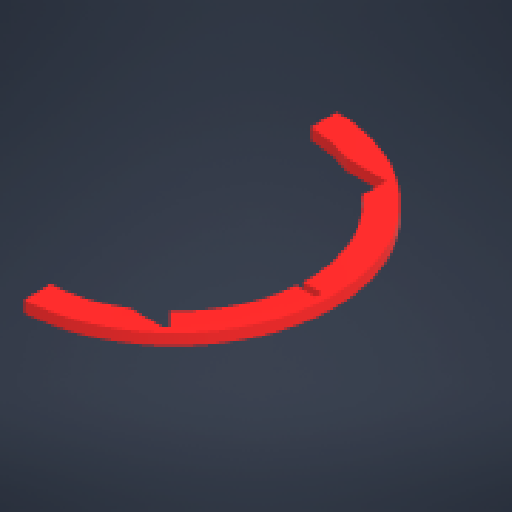
# Autodesk Inventor part: Back_front_aligner
Saved by Autodesk Inventor 2023 (Build 270158000, 158)
## iProperties
Created: 2023-05-09
Part Number: Back_front_aligner
Material: Generic
Document SubType Name: Modeling
Designer: szykr
Density: 1 g/cm^3
Appearance: Light Red
Author: szykr
Autodesk Inventor part; units mm, degrees
ref_plane "YZ Plane" through (0, 0, 0) normal (1, 0, 0) x (0, 1, 0)
ref_plane "XZ Plane" through (0, 0, 0) normal (0, 1, 0) x (-1, 0, 0)
ref_plane "XY Plane" through (0, 0, 0) normal (0, 0, 1) x (1, 0, 0)
sketch "Sketch1" plane through (0, 0, 0) normal (0, 1, 0) x (-1, 0, 0)
  circle A0 centre (0, 0) radius 40
  circle A1 centre (0, 0) radius 35
  line L0 (-0.75, -40) -> (-0.75, -35)
  line L1 (-23, -26.381812) -> (-23, -32.726136)
  line L2 (-34.93812, 2.828496) -> (-39.945867, 2.828496)
  line L3 (-39.945867, 1.33215) -> (-34.93812, 1.33215)
  line L4 (-24.132224, 25.315702) -> (-27.666452, 28.85856)
  line L5 (-26.660208, 29.866295) -> (-27.720868, 28.808219)
  line L6 (-39.940266, 2.933386) -> (-39.940266, 1.43704)
  line L7 (-23, -32.726136) -> (-21.5, -32.726136)
  circle A2 centre (0, 0) radius 42
  line L8 (-2.35, 40) -> (-2.35, 32.985933)
  line L9 (-27.666452, 28.85856) -> (-27.668423, 28.860536)
  line L10 (-26.660208, 29.866295) -> (-18.248408, 29.866295)
  line L11 (-21.5, -32.726136) -> (-12.409674, -32.726136)
  line L12 (-0.75, -35) -> (-0.75, -34.991963)
  line L13 (-34.93812, 2.828496) -> (-34.885522, 2.828496)
  line L14 (-39.945867, 1.33215) -> (-39.977811, 1.33215)
  line L15 (-39.940266, 1.43704) -> (-39.940266, 1.33215)
  line L16 (-0.75, -40) -> (-0.75, -41.993303)
  line L17 (-2.35, 40) -> (-2.35, 41.934204)
  line L18 (-39.892655, 2.928496) -> (-34.877269, 2.928496)
  line L19 (-34.978305, 1.23215) -> (-39.981018, 1.23215)
  line L20 (-39.892655, 2.928496) -> (-39.940266, 2.933386)
  point P0 (-24.149901, 25.333422)
  point P1 (-2.35, 34.921018)
  point P2 (-2.35, 39.930909)
  point P3 (-0.75, -39.992968)
  point P4 (-34.974639, 1.33215)
  point P5 (-39.89987, 2.828496)
  dimension "d0" = 2
  dimension "d3" = 0.1
  dimension "d4" = 0.1
  constraints: 24 end point, 5 point on circle, 4 collinear, 2 horizontal, 2 parallel, 2 point on line, 2 vertical, 1 centre point, 1 perpendicular, 7 other
  measures "d0" radial gap between concentric circles of A0 A2
  measures "d3" distance between parallel lines of L2 L18
  measures "d4" distance between parallel lines of L3 L19
sketch "Sketch1 outline for Extrusion1" plane through (0, 0, 0) normal (0, 1, 0) x (-1, 0, 0)
  line L0 (-27.666452, 28.85856) -> (-26.660208, 29.866295)
  line L1 (-24.149901, 25.333422) -> (-27.666452, 28.85856)
  arc A0 (-34.877269, 2.928496) -> (-24.149901, 25.333422) centre (0, 0) cw
  line L2 (-39.892655, 2.928496) -> (-34.877269, 2.928496)
  arc A1 (-39.981018, 1.23215) -> (-39.892655, 2.928496) centre (0, 0) cw
  line L3 (-34.978305, 1.23215) -> (-39.981018, 1.23215)
  arc A2 (-23, -26.381812) -> (-34.978305, 1.23215) centre (0, 0) cw
  line L4 (-23, -32.726136) -> (-23, -26.381812)
  line L5 (-21.5, -32.726136) -> (-23, -32.726136)
  line L6 (-12.409674, -32.726136) -> (-21.5, -32.726136)
  arc A3 (-0.75, -34.991963) -> (-12.409674, -32.726136) centre (0, 0) cw
  line L7 (-0.75, -35) -> (-0.75, -34.991963)
  line L8 (-0.75, -40) -> (-0.75, -35)
  line L9 (-0.75, -41.993303) -> (-0.75, -40)
  arc A4 (-2.35, 41.934204) -> (-0.75, -41.993303) centre (0, 0) ccw
  line L10 (-2.35, 40) -> (-2.35, 41.934204)
  line L11 (-2.35, 34.921018) -> (-2.35, 40)
  arc A5 (-18.248408, 29.866295) -> (-2.35, 34.921018) centre (0, 0) cw
  line L12 (-26.660208, 29.866295) -> (-18.248408, 29.866295)
extrude "Extrusion1" add sketch "Sketch1 outline for Extrusion1" along normal blind 3
equation "\"d4\" = slack"
equation "\"slack\" = 0.1"
body "Solid1"
